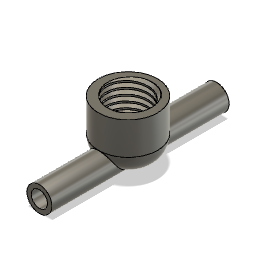
Inline Mic v4 (Autodesk Fusion 360 design; units mm, degrees)
Autodesk Fusion 360 part; units mm, degrees
note: some values were not read from the file. Set by a fixed rule: which face or edge a step refers to.
sketch "Sketch1" plane through (0, 0, 0) normal (0, 0, 1) x (1, 0, 0)
  circle A0 centre (0, 0) radius 4.25
  dimension "d1" = 8.5
  constraint coincident A0.centre origin
  measures "d1" diameter of A0
extrude "Extrude1" add sketch "Sketch1" along normal blind 40 makes body 1
ref_plane "WorkPlane1" through (0, 0, 20) normal (0, 0, -1) x (-1, 0, 0)
sketch "Sketch3" plane through (0, 0, 40) normal (0, 0, 1) x (1, 0, 0)
  circle A0 centre (0, 0) radius 4.25
  circle A1 centre (0, 0) radius 2.75
  dimension "d6" = 1.5
  constraint concentric A0 A1
  measures "d6" distance of A0 A1
sketch "Sketch4" plane through (0, 0, 20) normal (0, 0, -1) x (1, 0, 0)
  line L0 (-0.0035, 2.7336) -> (9.9965, 2.7336)
  line L1 (9.9965, 2.7336) -> (9.9965, -15.2664)
  line L2 (9.9965, -15.2664) -> (-0.0035, -15.2664)
  line L3 (-0.0035, -15.2664) -> (-0.0035, 2.7336)
  dimension "d7" = 10
  dimension "d8" = 18
  constraint horizontal L0
  constraint vertical L1
  constraint horizontal L2
  constraint vertical L3
  measures "d7" distance of L0.start L0.end
  measures "d8" distance of L0.start L2.end
revolve "Revolve1" add sketch "Sketch4" angle 360 about axis through (-0.0035, 15.2664, 20) along (0, -1, 0) separate body makes body 2
fillet "Fillet1" radius 7 1 edges at (-9.3268, -2.7336, 23.6162) on bodies 2
extrude "Extrude2" cut sketch "Sketch3" against normal up to surface (40 mm away) contours A1 bodies 1 2
sketch "Sketch5" plane through (0, 15.2664, 0) normal (0, 1, 0) x (-1, 0, 0)
  circle A0 centre (0.0035, 20) radius 10
  circle A1 centre (0.0035, 20) radius 8
  dimension "d13" = 16
  constraint concentric A0 A1
  measures "d13" diameter of A1
extrude "Extrude3" cut sketch "Sketch5" against normal blind 13.3 contours A1 bodies 1 2
extrude "Extrude4" add 2 faces at (-3.2555, 1.9664, 21.7943) (4.9591, 1.9664, 17.5342) along direction (0, 1, 0) blind 0.3 on bodies 2 bodies 2 1
thread "Thread1" "ISO Metric profile 16.0 M16x2 6H" major diameter 16.2505 minor diameter 14.0225 pitch 2 angle 60 modelled right hand crest width 0.5471 on face at (2.2113, 10.933, 27.6873) from (-0.0035, 15.2664, 20) to (-0.0035, 2.2664, 20) crest through (-7.0148, 14.7664, 20) on bodies 2
extrude "Extrude5" add 1 faces at (3.7239, -0.3478, 0) along direction (0, 0, -1) blind 10 on bodies 2 bodies 2
extrude "Extrude6" add 1 faces at (3.7239, -0.3478, 40) along direction (0, 0, 1) blind 10 on bodies 2 bodies 2
